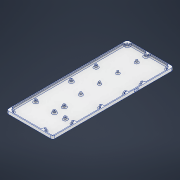
# Autodesk Inventor part: Base
Saved by Autodesk Inventor 2022 (Build 260153000, 153)
## iProperties
Created: 2021-09-21
Part Number: Base
Material: アルミニウム 6061
Document SubType Name: Modeling
Designer: shiok
Density: 2.7 g/cm^3
Appearance: アルミニウム - フラット
Author: shiok
Autodesk Inventor part; units mm, degrees
ref_plane "YZ Plane" through (0, 0, 0) normal (1, 0, 0) x (0, 1, 0)
ref_plane "XZ Plane" through (0, 0, 0) normal (0, 1, 0) x (-1, 0, 0)
ref_plane "XY Plane" through (0, 0, 0) normal (0, 0, 1) x (1, 0, 0)
ref_plane "作業平面5" through (0, 0, 0) normal (0, -1, 0) x (1, 0, 0)
sketch "スケッチ16" plane through (0, 0, 0) normal (0, -1, 0) x (1, 0, 0)
  line L0 (-65.12, -185.7375) -> (65.12, -185.7375)
  line L1 (71.12, -179.7375) -> (71.12, 179.7375)
  line L2 (65.12, 185.7375) -> (-65.12, 185.7375)
  line L3 (-71.12, 179.7375) -> (-71.12, -179.7375)
  arc A0 (-71.12, -179.7375) -> (-65.12, -185.7375) centre (-65.12, -179.7375) ccw
  arc A1 (65.12, -185.7375) -> (71.12, -179.7375) centre (65.12, -179.7375) ccw
  arc A2 (71.12, 179.7375) -> (65.12, 185.7375) centre (65.12, 179.7375) ccw
  arc A3 (-65.12, 185.7375) -> (-71.12, 179.7375) centre (-65.12, 179.7375) ccw
  line L4 (-65.12, -179.7375) -> (65.12, 179.7375)
  line L5 (-65.12, 179.7375) -> (65.12, -179.7375)
  point P0 (0, 0)
  point P1 (71.12, 185.7375)
  point P2 (71.12, -185.7375)
  point P3 (-71.12, 185.7375)
  point P4 (0, 0)
  point P5 (0, 0)
  dimension "d108" = 142.24
  dimension "d109" = 371.475
  dimension "d110" = 6
  constraints: 12 end point, 8 point on circle, 8 tangent, 6 point on line, 4 centre point, 3 equal radius, 3 midpoint, 2 parallel, 1 coincident, 1 horizontal, 1 perpendicular
  measures "d108" distance of point (-71.12, 185.738) point (71.12, 185.738)
  measures "d109" distance of point (71.12, 185.738) point (71.12, -185.738)
  measures "d110" radius of A0
extrude "押し出し12" add sketch "スケッチ16" against normal blind 2.6
sketch "スケッチ17" plane through (0, 2.6, 0) normal (0, 1, 0) x (1, 0, 0)
  line L0 (65.58, 183.1975) -> (-65.58, 183.1975)
  line L1 (-68.58, 180.1975) -> (-68.58, -180.1975)
  line L2 (-65.58, -183.1975) -> (65.58, -183.1975)
  line L3 (68.58, -180.1975) -> (68.58, 180.1975)
  arc A0 (68.58, 180.1975) -> (65.58, 183.1975) centre (65.58, 180.1975) ccw
  arc A1 (65.58, -183.1975) -> (68.58, -180.1975) centre (65.58, -180.1975) ccw
  arc A2 (-68.58, -180.1975) -> (-65.58, -183.1975) centre (-65.58, -180.1975) ccw
  arc A3 (-65.58, 183.1975) -> (-68.58, 180.1975) centre (-65.58, 180.1975) ccw
  line L4 (71.12, 180.1975) -> (71.12, -180.1975)
  arc A4 (65.58, -185.7375) -> (71.12, -180.1975) centre (65.58, -180.1975) ccw
  line L5 (65.58, -185.7375) -> (-65.58, -185.7375)
  arc A5 (-71.12, -180.1975) -> (-65.58, -185.7375) centre (-65.58, -180.1975) ccw
  line L6 (-71.12, -180.1975) -> (-71.12, 180.1975)
  arc A6 (-65.58, 185.7375) -> (-71.12, 180.1975) centre (-65.58, 180.1975) ccw
  line L7 (-65.58, 185.7375) -> (65.58, 185.7375)
  arc A7 (71.12, 180.1975) -> (65.58, 185.7375) centre (65.58, 180.1975) ccw
  line L8 (-65.58, 180.1975) -> (65.58, -180.1975) construction
  line L9 (-65.58, -180.1975) -> (65.58, 180.1975) construction
  circle A8 centre (62.23, 176.8475) radius 4
  circle A9 centre (63.5, 96.8375) radius 4
  circle A10 centre (63.5, 46.0375) radius 4
  circle A11 centre (62.23, -28.8925) radius 4
  circle A12 centre (62.23, -113.9825) radius 4
  circle A13 centre (38.1, -113.9825) radius 4
  circle A14 centre (38.1, -176.8475) radius 4
  circle A15 centre (-62.23, -176.8475) radius 4
  circle A16 centre (4.445, -113.9825) radius 4
  circle A17 centre (4.445, -83.5025) radius 4
  circle A18 centre (-52.705, -113.9825) radius 4
  circle A19 centre (-52.705, -4.7625) radius 4
  circle A20 centre (-52.705, 71.4375) radius 4
  circle A21 centre (-62.23, 176.8475) radius 4
  circle A22 centre (-5.08, 176.8475) radius 4
  point P0 (0, 0)
  point P1 (0, 0)
  point P2 (0, 0)
  point P3 (0, 0)
  point P4 (52.07, 166.6875)
  dimension "d113" = 3
  dimension "d114" = 2.54
  dimension "d115" = 366.395
  dimension "d116" = 137.16
  dimension "d117" = 16.51
  dimension "d118" = 16.51
  dimension "d119" = 10.16
  dimension "d120" = 10.16
  dimension "d121" = 1.27
  dimension "d122" = 1.27
  dimension "d123" = 80.01
  dimension "d124" = 50.8
  dimension "d125" = 74.93
  dimension "d126" = 85.09
  dimension "d127" = 8
  dimension "d128" = 8
  dimension "d129" = 8
  dimension "d130" = 8
  dimension "d131" = 8
  dimension "d132" = 24.13
  dimension "d133" = 62.865
  dimension "d134" = 100.33
  dimension "d135" = 62.865
  dimension "d136" = 9.525
  dimension "d137" = 8
  dimension "d138" = 8
  dimension "d139" = 57.15
  dimension "d140" = 76.2
  dimension "d141" = 8
  dimension "d142" = 8
  dimension "d143" = 109.22
  dimension "d144" = 8
  dimension "d145" = 8
  dimension "d146" = 8
  dimension "d147" = 8
  dimension "d148" = 8
  dimension "d149" = 8
  dimension "d150" = 30.48
  dimension "d151" = 33.655
  constraints: 23 centre point, 20 end point, 16 point on circle, 8 tangent, 7 vertical alignment, 5 horizontal alignment, 4 parallel, 3 equal radius, 3 midpoint, 2 perpendicular, 1 coincident, 1 horizontal, 7 other
  measures "d113" radius of A0
  measures "d114" distance between parallel lines of L3 L4
  measures "d115" distance between parallel lines of L2 L0
  measures "d116" distance between parallel lines of L1 L3
  measures "d117" distance from line of point (52.07, 166.688) L3
  measures "d118" distance from line of L0 point (52.07, 166.688)
  measures "d119" horizontal distance of A8.centre point (52.07, 166.688)
  measures "d120" horizontal distance of point (52.07, 166.688) A8.centre
  measures "d121" horizontal distance of A9.centre A8.centre
  measures "d122" horizontal distance of A11.centre A10.centre
  measures "d123" vertical distance of A9.centre A8.centre
  measures "d124" distance of A9.centre A10.centre
  measures "d125" vertical distance of A10.centre A11.centre
  measures "d126" distance of A12.centre A11.centre
  measures "d127" diameter of A8
  measures "d128" diameter of A9
  measures "d129" diameter of A10
  measures "d130" diameter of A11
  measures "d131" diameter of A12
  measures "d132" distance of A13.centre A12.centre
  measures "d133" distance of A14.centre A13.centre
  measures "d134" distance of A15.centre A14.centre
  measures "d135" vertical distance of A18.centre A15.centre
  measures "d136" horizontal distance of A18.centre A15.centre
  measures "d137" diameter of A21
  measures "d138" diameter of A22
  measures "d139" distance of A21.centre A22.centre
  measures "d140" distance of A19.centre A20.centre
  measures "d141" diameter of A20
  measures "d142" diameter of A19
  measures "d143" distance of A18.centre A19.centre
  measures "d144" diameter of A13
  measures "d145" diameter of A14
  measures "d146" diameter of A15
  measures "d147" diameter of A18
  measures "d148" diameter of A17
  measures "d149" diameter of A16
  measures "d150" distance of A17.centre A16.centre
  measures "d151" distance of A13.centre A16.centre
extrude "押し出し13" add sketch "スケッチ17" along normal blind 6.4 and the other way blind 3 contours A8 | A9 | A10 | A11 | A12 | A13 | A14 | A15 | A16 | A17 | A18 | A19 | A20 | A21 | A22
sketch "スケッチ18" plane through (0, 2.6, 0) normal (0, 1, 0) x (1, 0, 0)
  line L0 (-65.12, -185.7375) -> (65.12, -185.7375)
  line L1 (71.12, -179.7375) -> (71.12, 179.7375)
  line L2 (65.12, 185.7375) -> (-65.12, 185.7375)
  line L3 (-71.12, 179.7375) -> (-71.12, -179.7375)
  arc A0 (-71.12, -179.7375) -> (-65.12, -185.7375) centre (-65.12, -179.7375) ccw
  arc A1 (65.12, -185.7375) -> (71.12, -179.7375) centre (65.12, -179.7375) ccw
  arc A2 (71.12, 179.7375) -> (65.12, 185.7375) centre (65.12, 179.7375) ccw
  arc A3 (-65.12, 185.7375) -> (-71.12, 179.7375) centre (-65.12, 179.7375) ccw
  line L4 (-65.12, -179.7375) -> (65.12, 179.7375)
  line L5 (-65.12, 179.7375) -> (65.12, -179.7375)
  line L6 (68.58, 179.7375) -> (68.58, -179.7375)
  arc A4 (65.12, -183.1975) -> (68.58, -179.7375) centre (65.12, -179.7375) ccw
  line L7 (65.12, -183.1975) -> (-65.12, -183.1975)
  arc A5 (-68.58, -179.7375) -> (-65.12, -183.1975) centre (-65.12, -179.7375) ccw
  line L8 (-68.58, -179.7375) -> (-68.58, 179.7375)
  arc A6 (-65.12, 183.1975) -> (-68.58, 179.7375) centre (-65.12, 179.7375) ccw
  line L9 (-65.12, 183.1975) -> (65.12, 183.1975)
  arc A7 (68.58, 179.7375) -> (65.12, 183.1975) centre (65.12, 179.7375) ccw
  point P0 (0, 0)
  point P1 (0, 0)
  point P2 (71.12, 185.7375)
  point P3 (71.12, -185.7375)
  point P4 (-71.12, 185.7375)
  point P5 (0, 0)
  point P6 (0, 0)
  dimension "d154" = 142.24
  dimension "d155" = 371.475
  dimension "d156" = 6
  dimension "d157" = 2.54
  constraints: 20 end point, 16 point on circle, 8 centre point, 8 tangent, 6 point on line, 4 parallel, 3 equal radius, 3 midpoint, 2 perpendicular, 1 coincident, 1 horizontal, 7 other
  measures "d154" distance of point (-71.12, 185.738) point (71.12, 185.738)
  measures "d155" distance of point (71.12, 185.738) point (71.12, -185.738)
  measures "d156" radius of A0
  measures "d157" distance between parallel lines of L1 L6
extrude "押し出し14" add sketch "スケッチ18" along normal blind 6.4
sketch "スケッチ20" plane through (-5.08, 9, -176.8475) normal (0, 1, 0) x (1, 0, 0)
  line L0 (1.78, -7.62) -> (1.78, -260.35)
  circle A0 centre (1.78, -29.97) radius 3
  circle A1 centre (1.78, -87.88) radius 2.5
  circle A2 centre (1.78, -144.27) radius 2.5
  circle A3 centre (1.78, -201.67) radius 3
  point P0 (5.08, -176.8475)
  point P1 (0, 0)
  point P2 (0, 0)
  dimension "d167" = 1.78
  dimension "d218" = 6
  dimension "d219" = 5
  dimension "d220" = 5
  dimension "d221" = 6
  dimension "d222" = 57.91
  dimension "d223" = 29.97
  dimension "d224" = 56.39
  dimension "d225" = 57.4
  constraints: 4 centre point, 4 point on line, 2 end point, 1 coincident, 1 vertical, 1 other
  measures "d167" distance from line of point (0, 0) L0
  measures "d218" diameter of A0
  measures "d219" diameter of A1
  measures "d220" diameter of A2
  measures "d221" diameter of A3
  measures "d222" distance of A0.centre A1.centre
  measures "d223" vertical distance of point (0, 0) A0.centre
  measures "d224" distance of A2.centre A1.centre
  measures "d225" distance of A3.centre A2.centre
extrude "押し出し15" add sketch "スケッチ20" against normal up to surface (6.4 mm away)
sketch "スケッチ21" plane through (71.12, 0, 179.7375) normal (1, 0, 0) x (0, 0, -1)
  line L0 (244.682, 7.6) -> (257.682, 7.6)
  line L1 (257.682, 7.6) -> (257.682, 2.6)
  line L2 (257.682, 2.6) -> (244.682, 2.6)
  line L3 (244.682, 2.6) -> (244.682, 7.6)
  line L4 (365.475, 0) -> (365.475, 9) projected
  line L5 (359.475, 0) -> (0, 0) projected
  point P0 (179.7375, 0)
  dimension "d171" = 13
  dimension "d172" = 5
  dimension "d173" = 107.793
  dimension "d174" = 2.6
  constraints: 8 end point, 2 parallel, 1 horizontal, 1 perpendicular
  measures "d171" distance of L1.end L2.end
  measures "d172" distance of L0.end L1.end
  measures "d173" distance between parallel lines of L4 L1
  measures "d174" distance between parallel lines of L5 L2
extrude "押し出し16" cut sketch "スケッチ21" against normal blind 10
fillet "フィレット8" radius 2.5 4 edges at (69.85, 2.6, -64.9445) (69.85, 2.6, -77.9445) (69.85, 7.6, -64.9445) (69.85, 7.6, -77.9445)
sketch "スケッチ23" plane through (0, 0, 0) normal (0, -1, 0) x (1, 0, 0)
  point P0 (0, 0)
sketch "スケッチ24" plane through (0, 9, 0) normal (0, 1, 0) x (1, 0, 0)
  line L0 (62.23, 172.8475) -> (69.1721, 172.8475)
  line L1 (69.1721, 172.8475) -> (69.1721, 183.2244)
  line L2 (69.1721, 183.2244) -> (58.23, 183.2244)
  line L3 (58.23, 183.2244) -> (58.23, 176.8475)
  line L4 (69.9236, 100.8375) -> (63.5, 100.8375)
  line L5 (63.5, 92.8375) -> (69.9236, 92.8375)
  line L6 (69.9236, 92.8375) -> (69.9236, 100.8375)
  line L7 (69.9236, 50.0375) -> (63.5, 50.0375)
  line L8 (63.5, 42.0375) -> (69.9236, 42.0375)
  line L9 (69.9236, 42.0375) -> (69.9236, 50.0375)
  line L10 (69.9236, -24.8925) -> (62.23, -24.8925)
  line L11 (62.23, -32.8925) -> (69.9236, -32.8925)
  line L12 (69.9236, -32.8925) -> (69.9236, -24.8925)
  line L13 (69.9236, -109.9825) -> (62.23, -109.9825)
  line L14 (62.23, -117.9825) -> (69.9236, -117.9825)
  line L15 (69.9236, -117.9825) -> (69.9236, -109.9825)
  line L16 (42.1, -185.0496) -> (34.1, -185.0496)
  line L17 (34.1, -185.0496) -> (34.1, -176.8475)
  line L18 (42.1, -176.8475) -> (42.1, -185.0496)
  line L19 (-69.2508, -183.7021) -> (-58.23, -183.7021)
  line L20 (-58.23, -183.7021) -> (-58.23, -176.8475)
  line L21 (-62.23, -172.8475) -> (-69.2508, -172.8475)
  line L22 (-69.2508, -172.8475) -> (-69.2508, -183.7021)
  line L23 (-62.23, 172.8475) -> (-69.1412, 172.8475)
  line L24 (-69.1412, 172.8475) -> (-69.1412, 183.2244)
  line L25 (-69.1412, 183.2244) -> (-58.23, 183.2244)
  line L26 (-58.23, 183.2244) -> (-58.23, 176.8475)
  line L27 (-1.08, 184.7805) -> (-9.08, 184.7805)
  line L28 (-9.08, 184.7805) -> (-9.08, 176.8475)
  line L29 (-1.08, 176.8475) -> (-1.08, 184.7805)
  circle A0 centre (62.23, 176.8475) radius 4 projected
  circle A1 centre (63.5, 96.8375) radius 4 projected
  circle A2 centre (63.5, 46.0375) radius 4 projected
  circle A3 centre (62.23, -28.8925) radius 4 projected
  circle A4 centre (62.23, -113.9825) radius 4 projected
  circle A5 centre (38.1, -176.8475) radius 4 projected
  circle A6 centre (-62.23, -176.8475) radius 4 projected
  circle A7 centre (-62.23, 176.8475) radius 4 projected
  circle A8 centre (-5.08, 176.8475) radius 4 projected
  point P0 (0, 0)
  constraints: 60 end point, 18 point on circle, 18 tangent, 12 parallel, 9 horizontal, 5 perpendicular, 4 point on line
extrude "押し出し17" add sketch "スケッチ24" against normal up to surface (9 mm away) from surface at 0 contours A0 L3 L2 L1 L0 | L6 L5 A1 L4 | L9 L8 A2 L7 | L12 L11 A3 L10 | L15 L14 A4 L13 | L16 L17 A5 L18 | L22 L21 A6 L20 L19 | L23 L24 L25 L26 A7 | L29 A8 L28 L27
sketch "スケッチ28" plane through (0, 2.6, 0) normal (0, 1, 0) x (1, 0, 0)
  circle A0 centre (62.23, 176.8475) radius 4
  arc A1 (68.58, 180.1975) -> (65.58, 183.1975) centre (65.58, 180.1975) ccw
  arc A2 (71.12, 180.1975) -> (65.58, 185.7375) centre (65.58, 180.1975) ccw
  circle A3 centre (-5.08, 176.8475) radius 4
  line L0 (65.58, 183.1975) -> (-65.58, 183.1975)
  line L1 (-65.58, 185.7375) -> (65.58, 185.7375)
  circle A4 centre (-62.23, 176.8475) radius 4
  arc A5 (-65.58, 183.1975) -> (-68.58, 180.1975) centre (-65.58, 180.1975) ccw
  arc A6 (-65.58, 185.7375) -> (-71.12, 180.1975) centre (-65.58, 180.1975) ccw
  circle A7 centre (63.5, 46.0375) radius 4
  circle A8 centre (63.5, 96.8375) radius 4
  line L2 (71.12, 180.1975) -> (71.12, -180.1975)
  line L3 (68.58, -180.1975) -> (68.58, 180.1975)
  line L4 (-65.58, 180.1975) -> (65.58, -180.1975) construction
  line L5 (-65.58, -180.1975) -> (65.58, 180.1975) construction
  line L6 (-71.12, -180.1975) -> (-71.12, 180.1975)
  line L7 (-68.58, 180.1975) -> (-68.58, -180.1975)
  circle A9 centre (-52.705, -4.7625) radius 4
  circle A10 centre (-52.705, 71.4375) radius 4
  line L8 (-65.58, -183.1975) -> (65.58, -183.1975)
  arc A11 (65.58, -183.1975) -> (68.58, -180.1975) centre (65.58, -180.1975) ccw
  arc A12 (-68.58, -180.1975) -> (-65.58, -183.1975) centre (-65.58, -180.1975) ccw
  arc A13 (65.58, -185.7375) -> (71.12, -180.1975) centre (65.58, -180.1975) ccw
  line L9 (65.58, -185.7375) -> (-65.58, -185.7375)
  arc A14 (-71.12, -180.1975) -> (-65.58, -185.7375) centre (-65.58, -180.1975) ccw
  circle A15 centre (4.445, -83.5025) radius 4
  circle A16 centre (62.23, -113.9825) radius 4
  circle A17 centre (38.1, -113.9825) radius 4
  circle A18 centre (4.445, -113.9825) radius 4
  circle A19 centre (-52.705, -113.9825) radius 4
  circle A20 centre (-62.23, -176.8475) radius 4
  circle A21 centre (38.1, -176.8475) radius 4
  circle A22 centre (62.23, -28.8925) radius 4
  point P0 (0, 0)
  point P1 (0, 0)
  point P2 (0, 0)
  point P3 (0, 0)
  point P4 (0, 0)
  point P5 (52.07, 166.6875)
  dimension "d308" = 3
  dimension "d309" = 2.54
  dimension "d310" = 366.395
  dimension "d311" = 137.16
  dimension "d312" = 16.51
  dimension "d313" = 16.51
  dimension "d314" = 10.16
  dimension "d315" = 10.16
  dimension "d316" = 1.27
  dimension "d317" = 1.27
  dimension "d318" = 80.01
  dimension "d319" = 50.8
  dimension "d320" = 74.93
  dimension "d321" = 85.09
  dimension "d322" = 8
  dimension "d323" = 8
  dimension "d324" = 8
  dimension "d325" = 8
  dimension "d326" = 8
  dimension "d327" = 24.13
  dimension "d328" = 62.865
  dimension "d329" = 100.33
  dimension "d330" = 62.865
  dimension "d331" = 9.525
  dimension "d332" = 8
  dimension "d333" = 8
  dimension "d334" = 57.15
  dimension "d335" = 76.2
  dimension "d336" = 8
  dimension "d337" = 8
  dimension "d338" = 109.22
  dimension "d339" = 8
  dimension "d340" = 8
  dimension "d341" = 8
  dimension "d342" = 8
  dimension "d343" = 8
  dimension "d344" = 8
  dimension "d345" = 30.48
  dimension "d346" = 33.655
  constraints: 23 centre point, 20 end point, 16 point on circle, 8 tangent, 7 vertical alignment, 5 horizontal alignment, 4 parallel, 3 equal radius, 3 midpoint, 2 perpendicular, 1 coincident, 1 horizontal, 7 other
  measures "d308" radius of A1
  measures "d309" distance between parallel lines of L3 L2
  measures "d310" distance between parallel lines of L8 L0
  measures "d311" distance between parallel lines of L7 L3
  measures "d312" distance from line of point (52.07, 166.688) L3
  measures "d313" distance from line of L0 point (52.07, 166.688)
  measures "d314" horizontal distance of A0.centre point (52.07, 166.688)
  measures "d315" horizontal distance of point (52.07, 166.688) A0.centre
  measures "d316" horizontal distance of A8.centre A0.centre
  measures "d317" horizontal distance of A22.centre A7.centre
  measures "d318" vertical distance of A8.centre A0.centre
  measures "d319" distance of A8.centre A7.centre
  measures "d320" vertical distance of A7.centre A22.centre
  measures "d321" distance of A16.centre A22.centre
  measures "d322" diameter of A0
  measures "d323" diameter of A8
  measures "d324" diameter of A7
  measures "d325" diameter of A22
  measures "d326" diameter of A16
  measures "d327" distance of A17.centre A16.centre
  measures "d328" distance of A21.centre A17.centre
  measures "d329" distance of A20.centre A21.centre
  measures "d330" vertical distance of A19.centre A20.centre
  measures "d331" horizontal distance of A19.centre A20.centre
  measures "d332" diameter of A4
  measures "d333" diameter of A3
  measures "d334" distance of A4.centre A3.centre
  measures "d335" distance of A9.centre A10.centre
  measures "d336" diameter of A10
  measures "d337" diameter of A9
  measures "d338" distance of A19.centre A9.centre
  measures "d339" diameter of A17
  measures "d340" diameter of A21
  measures "d341" diameter of A20
  measures "d342" diameter of A19
  measures "d343" diameter of A15
  measures "d344" diameter of A18
  measures "d345" distance of A15.centre A18.centre
  measures "d346" distance of A17.centre A18.centre
sketch "スケッチ32" plane through (38.1, -0.4, 176.8475) normal (0, -1, 0) x (1, 0, 0)
  point P0 (-38.1, -176.8475)
  point P1 (0, 0)
sketch "スケッチ33" plane through (38.1, -0.4, 113.9825) normal (0, -1, 0) x (1, 0, 0)
  circle A0 centre (0, 0) radius 4 projected
  point P0 (-38.1, -113.9825)
  constraints: 1 coincident
sketch "スケッチ34" plane through (62.23, -0.4, 113.9825) normal (0, -1, 0) x (1, 0, 0)
  point P0 (-62.23, -113.9825)
  point P1 (0, 0)
sketch "スケッチ35" plane through (62.23, -0.4, 28.8925) normal (0, -1, 0) x (1, 0, 0)
  point P0 (-62.23, -28.8925)
  point P1 (0, 0)
sketch "スケッチ36" plane through (63.5, -0.4, -46.0375) normal (0, -1, 0) x (1, 0, 0)
  point P0 (-63.5, 46.0375)
  point P1 (0, 0)
sketch "スケッチ37" plane through (63.5, -0.4, -96.8375) normal (0, -1, 0) x (1, 0, 0)
  point P0 (-63.5, 96.8375)
  point P1 (0, 0)
sketch "スケッチ38" plane through (62.23, -0.4, -176.8475) normal (0, -1, 0) x (1, 0, 0)
  point P0 (-62.23, 176.8475)
  point P1 (0, 0)
sketch "スケッチ39" plane through (-5.08, -0.4, -176.8475) normal (0, -1, 0) x (1, 0, 0)
  point P0 (5.08, 176.8475)
sketch "スケッチ40" plane through (-5.08, -0.4, -176.8475) normal (0, -1, 0) x (1, 0, 0)
  arc A0 (4, 0) -> (-4, 0) centre (0, 0) ccw projected
  point P0 (5.08, 176.8475)
  constraints: 1 coincident
sketch "スケッチ41" plane through (-62.23, -0.4, -176.8475) normal (0, -1, 0) x (1, 0, 0)
  circle A0 centre (0, 0) radius 4 projected
  point P0 (62.23, 176.8475)
  constraints: 1 coincident
sketch "スケッチ42" plane through (-52.705, -0.4, -71.4375) normal (0, -1, 0) x (1, 0, 0)
  circle A0 centre (0, 0) radius 4 projected
  point P0 (52.705, 71.4375)
  constraints: 1 coincident
sketch "スケッチ43" plane through (-52.705, -0.4, 4.7625) normal (0, -1, 0) x (1, 0, 0)
  circle A0 centre (0, 0) radius 4 projected
  point P0 (52.705, -4.7625)
  constraints: 1 coincident
sketch "スケッチ44" plane through (4.445, -0.4, 83.5025) normal (0, -1, 0) x (1, 0, 0)
  circle A0 centre (0, 0) radius 4 projected
  point P0 (-4.445, -83.5025)
  constraints: 1 coincident
sketch "スケッチ45" plane through (4.445, -0.4, 113.9825) normal (0, -1, 0) x (1, 0, 0)
  circle A0 centre (0, 0) radius 4 projected
  point P0 (-4.445, -113.9825)
  constraints: 1 coincident
sketch "スケッチ46" plane through (-52.705, -0.4, 113.9825) normal (0, -1, 0) x (1, 0, 0)
  point P0 (52.705, -113.9825)
  point P1 (0, 0)
  point P2 (0, 0)
  constraints: 1 coincident
sketch "スケッチ47" plane through (-62.23, -0.4, 176.8475) normal (0, -1, 0) x (1, 0, 0)
  point P0 (62.23, -176.8475)
  point P1 (0, 0)
hole "穴1" at (38.1, -0.4, 176.8475) direction (0, 1, 0) diameter 3.4 end through all counterbore diameter 6 counterbore depth 4.46
hole "穴2" at (38.1, -0.4, 113.9825) direction (0, 1, 0) diameter 3.4 end through all counterbore diameter 6 counterbore depth 4.46
hole "穴3" at (62.23, -0.4, 113.9825) direction (0, 1, 0) diameter 3.4 end through all counterbore diameter 6 counterbore depth 4.46
hole "穴4" at (62.23, -0.4, 28.8925) direction (0, 1, 0) diameter 3.4 end through all counterbore diameter 6 counterbore depth 4.46
hole "穴5" at (63.5, -0.4, -46.0375) direction (0, 1, 0) diameter 3.4 end through all counterbore diameter 6 counterbore depth 4.46
hole "穴6" at (63.5, -0.4, -96.8375) direction (0, 1, 0) diameter 3.4 end through all counterbore diameter 6 counterbore depth 4.46
hole "穴7" at (4.445, -0.4, 113.9825) direction (0, 1, 0) diameter 3.4 end through all counterbore diameter 6 counterbore depth 4.46
hole "穴8" at (4.445, -0.4, 83.5025) direction (0, 1, 0) diameter 3.4 end through all counterbore diameter 6 counterbore depth 4.46
hole "穴9" at (62.23, -0.4, -176.8475) direction (0, 1, 0) diameter 3.4 end through all counterbore diameter 6 counterbore depth 4.46
hole "穴10" at (-5.08, -0.4, -176.8475) direction (0, 1, 0) diameter 3.4 end through all counterbore diameter 6 counterbore depth 4.46
hole "穴11" at (-62.23, -0.4, -176.8475) direction (0, 1, 0) diameter 3.4 end through all counterbore diameter 6 counterbore depth 4.46
hole "穴12" at (-52.705, -0.4, -71.4375) direction (0, 1, 0) diameter 3.4 end through all counterbore diameter 6 counterbore depth 4.46
hole "穴13" at (-52.705, -0.4, 4.7625) direction (0, 1, 0) diameter 3.4 end through all counterbore diameter 6 counterbore depth 4.46
hole "穴14" at (-52.705, -0.4, 113.9825) direction (0, 1, 0) diameter 3.4 end through all counterbore diameter 6 counterbore depth 4.46
hole "穴15" at (-62.23, -0.4, 176.8475) direction (0, 1, 0) diameter 3.4 end through all counterbore diameter 6 counterbore depth 4.46
fillet "フィレット13" radius 3 50 edges at (-12.065, 2.6, 183.1975) (-68.58, 2.6, 0) (-65.405, 2.6, -172.8475) (-58.23, 2.6, -180.0225) (-59.4016, 2.6, -174.0191) (-33.655, 2.6, -183.1975) (-9.08, 2.6, -180.0225) (-1.08, 2.6, -180.0225) (-5.08, 2.6, -172.8475) (28.575, 2.6, -183.1975) (58.23, 2.6, -180.0225) (65.405, 2.6, -172.8475) (59.4016, 2.6, -174.0191) (68.58, 2.6, -136.8425) (66.04, 2.6, -100.8375) (66.04, 2.6, -92.8375) (59.5, 2.6, -96.8375) (68.58, 2.6, -84.1411) (68.58, 2.6, -58.741) (59.5, 2.6, -46.0375) (66.04, 2.6, -42.0375) (66.04, 2.6, -50.0375) (68.58, 2.6, -8.5725) (58.23, 2.6, 28.8925) (65.405, 2.6, 32.8925) (65.405, 2.6, 24.8925) (68.58, 2.6, 71.4375) (58.23, 2.6, 113.9825) (65.405, 2.6, 117.9825) (65.405, 2.6, 109.9825) (67.5666, 2.6, 182.1841) (53.61, 2.6, 183.1975) (68.58, 2.6, 148.86) (42.1, 2.6, 180.0225) (34.1, 2.6, 180.0225) (38.1, 2.6, 172.8475) (-58.23, 2.6, 180.0225) (-65.405, 2.6, 172.8475) (-59.4016, 2.6, 174.0191) (58.23, 5.8, -183.1975) (68.58, 5.8, -172.8475) (-1.08, 5.8, -183.1975) (-9.08, 5.8, -183.1975) (-58.23, 5.8, -183.1975) (-68.58, 5.8, -172.8475) (-68.58, 5.8, 172.8475) (-58.23, 5.8, 183.1975) (34.1, 5.8, 183.1975) (42.1, 5.8, 183.1975) (68.58, 5.8, 117.9825)
fillet "フィレット14" radius 3 14 edges at (67.7013, 3.4787, 109.1038) (68.58, 7.3, 109.9825) (67.7013, 3.4787, 33.7712) (68.58, 7.3, 32.8925) (67.7013, 3.4787, 24.0138) (68.58, 7.3, 24.8925) (68.58, 7.3, -50.0375) (67.7013, 3.4787, -50.9162) (67.7013, 3.4787, -101.7162) (68.58, 7.3, -100.8375) (67.7013, 3.4787, -91.9588) (68.58, 7.3, -92.8375) (67.7013, 3.4787, -41.1588) (68.58, 7.3, -42.0375)
sketch "スケッチ48" plane through (0, 0, 0) normal (0, -1, 0) x (1, 0, 0)
  line L0 (-87.5908, -211.4867) -> (95.1488, -211.4867)
  line L1 (95.1488, -211.4867) -> (95.1488, 206.898)
  line L2 (95.1488, 206.898) -> (-87.5908, 206.898)
  line L3 (-87.5908, 206.898) -> (-87.5908, -211.4867)
  point P0 (0, 0)
  constraints: 8 end point, 2 parallel, 1 horizontal, 1 perpendicular
extrude "押し出し18" cut sketch "スケッチ48" along normal up to surface (0.4 mm away) from surface at 0
fillet "フィレット15" radius 3 10 edges at (-56.705, 2.6, 113.9825) (-56.705, 2.6, 4.7625) (-56.705, 2.6, -71.4375) (-6.3, 2.6, -146.8775) (-5.8, 2.6, -88.9675) (-5.8, 2.6, -32.5775) (-6.3, 2.6, 24.8225) (0.445, 2.6, 83.5025) (0.445, 2.6, 113.9825) (34.1, 2.6, 113.9825)
